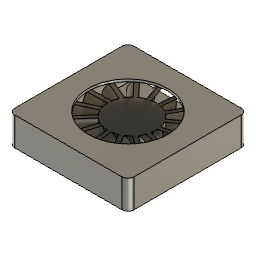
JMS583硬盘盒外壳 (Autodesk Fusion 360 archive; units mm, degrees)
design "3007涡轮风扇"
Autodesk Fusion 360 part; units mm, degrees
note: some values were not read from the file. Chosen so that the rebuilt part matches the saved one: which face or edge a step refers to; where a step ends.
box "长方体基本要素1" add length 30 width 30 height 7.2 placed x (0, 1, 0) y (-1, 0, 0) z (0, 0, 1) at (30, 0, 0) makes body 1
fillet "圆角1" radius 1.5 4 edges at (0, 0, 3.6) (30, 0, 3.6) (30, 30, 3.6) (0, 30, 3.6) on bodies 1
sketch "草图2" plane through (0, 30, 0) normal (0, 1, 0) x (-1, 0, 0)
  line L0 (-1.5, 0) -> (-1.5, 7.2)
  line L1 (-1.5, 7.2) -> (-28.5, 7.2)
  line L2 (-28.5, 7.2) -> (-28.5, 0)
  line L3 (-28.5, 0) -> (-1.5, 0)
  line L4 (-27.9, 0.6) -> (-2.1, 0.6)
  line L5 (-2.1, 0.6) -> (-2.1, 6.6)
  line L6 (-2.1, 6.6) -> (-27.9, 6.6)
  line L7 (-27.9, 6.6) -> (-27.9, 0.6)
  dimension "d10" = -0.6
extrude "拉伸1" cut sketch "草图2" against normal blind 28 contours L4 L5 L6 L7 bodies 1
sketch "草图3" plane through (0, 0, 7.2) normal (0, 0, 1) x (-1, 0, 0)
  arc A0 (-1.5, -30) -> (0, -28.5) centre (-1.5, -28.5) ccw
  line L0 (0, -28.5) -> (0, -1.5)
  arc A1 (0, -1.5) -> (-1.5, 0) centre (-1.5, -1.5) ccw
  line L1 (-1.5, 0) -> (-28.5, 0)
  arc A2 (-28.5, 0) -> (-30, -1.5) centre (-28.5, -1.5) ccw
  line L2 (-30, -1.5) -> (-30, -28.5)
  arc A3 (-30, -28.5) -> (-28.5, -30) centre (-28.5, -28.5) ccw
  line L3 (-28.5, -30) -> (-1.5, -30)
  circle A4 centre (-15, -15) radius 10
  dimension "d13" = 20
  measures "d13" diameter of A4
extrude "拉伸2" cut sketch "草图3" against normal up to surface (0.6 mm away) contours A4 bodies 1
sketch "草图4" plane through (0, 0, 0.6) normal (0, 0, 1) x (-1, 0, 0)
  line L0 (-27.9, -30) -> (-2.1, -30)
  line L1 (-2.1, -30) -> (-2.1, -2)
  line L2 (-2.1, -2) -> (-27.9, -2)
  line L3 (-27.9, -2) -> (-27.9, -30)
  circle A0 centre (-15, -15) radius 6
  dimension "d16" = 12
  measures "d16" diameter of A0
extrude "拉伸3" add sketch "草图4" along normal blind 5 separate body contours A0 makes body 2
ref_plane "工作平面1" through (15, 21, 3.0297) normal (0, 1, 0) x (1, 0, 0)
sketch "草图5" plane through (0, 21, 0) normal (0, 1, 0) x (1, 0, 0)
  line L0 (15, -7.5) -> (15, 2.5) construction
  spline S0 degree 5 poles (15, -5.6) (14.9831, -5.5891) (14.9491, -5.5667) (14.8976, -5.5318) (14.8282, -5.4822) (14.7402, -5.4155) (14.6512, -5.344) (14.5618, -5.2681) (14.473, -5.1883) (14.3862, -5.1053) (14.3029, -5.0196) (14.2243, -4.9315) (14.1513, -4.8408) (14.0838, -4.7462) (14.0213, -4.6459) (13.9629, -4.5383) (13.9079, -4.4221) (13.8562, -4.2971) (13.8086, -4.1649) (13.7665, -4.0281) (13.7316, -3.8896) (13.7053, -3.7523) (13.6885, -3.6176) (13.681, -3.4853) (13.6813, -3.3535) (13.6872, -3.2193) (13.696, -3.0801) (13.7041, -2.9338) (13.7079, -2.7799) (13.7037, -2.62) (13.6884, -2.4567) (13.6593, -2.2933) (13.6154, -2.1333) (13.557, -1.9799) (13.4868, -1.8355) (13.4089, -1.7015) (13.3279, -1.5784) (13.2483, -1.466) (13.1736, -1.3637) (13.1048, -1.2698) (13.0409, -1.1824) (12.9792, -1.0993) (12.9162, -1.0185) (12.8489, -0.9379) (12.7748, -0.8565) (12.6927, -0.7733) (12.62, -0.7051) (12.5616, -0.6529) (12.5208, -0.6177) (12.5, -0.6) knots 0 0 0 0 0 0 0.022222 0.044444 0.066667 0.088889 0.111111 0.133333 0.155556 0.177778 0.2 0.222222 0.244444 0.266667 0.288889 0.311111 0.333333 0.355556 0.377778 0.4 0.422222 0.444444 0.466667 0.488889 0.511111 0.533333 0.555556 0.577778 0.6 0.622222 0.644444 0.666667 0.688889 0.711111 0.733333 0.755556 0.777778 0.8 0.822222 0.844444 0.866667 0.888889 0.911111 0.933333 0.955556 0.977778 1 1 1 1 1 1
  spline S1 degree 3 poles (15.271, -5.1798) (15.0406, -5.0312) (14.7397, -4.7805) (14.5633, -4.5536) (14.4521, -4.4106) (14.3637, -4.2419) (14.2867, -4.0127) (14.217, -3.8056) (14.1821, -3.6167) (14.182, -3.4179) (14.1818, -3.1927) (14.2371, -2.8509) (14.1851, -2.4258) (14.1364, -2.027) (13.9458, -1.6066) (13.7657, -1.3356) (13.5507, -1.0121) (13.4347, -0.8538) (13.2399, -0.6274) (13.1243, -0.493) (12.9854, -0.3565) (12.824, -0.2192) knots 0 0 0 0 0.21724 0.21724 0.21724 0.354174 0.354174 0.354174 0.477946 0.477946 0.477946 0.618157 0.618157 0.618157 0.749718 0.749718 0.749718 0.906788 0.906788 0.906788 1 1 1 1
  spline S2 degree 5 poles (15.271, -5.1798) (15.2763, -5.1878) (15.2879, -5.2041) (15.3088, -5.229) (15.3435, -5.2633) (15.3989, -5.308) (15.4662, -5.3542) (15.5448, -5.4012) (15.6307, -5.447) (15.7206, -5.4902) (15.8127, -5.5302) (15.8872, -5.5597) (15.9435, -5.5804) (15.9811, -5.5936) (16, -5.6) knots 0 0 0 0 0 0 0.1 0.2 0.3 0.4 0.5 0.6 0.7 0.8 0.9 1 1 1 1 1 1
  line L1 (15.453, -5.3473) -> (15.6179, -5.4418)
  line L2 (16, -5.6) -> (15, -5.6)
  line L3 (12.5, -0.6) -> (13.2161, -0.6)
  point P0 (14.6, -5.3)
  point P1 (14.2, -4.9)
  point P2 (13.9, -4.4)
  point P3 (13.7, -3.7)
  point P4 (13.7, -3)
  point P5 (13.6, -2.1)
  point P6 (13.2, -1.4)
  point P7 (12.9, -1)
  point P8 (15.5354, -5.3945)
  dimension "d21" = 0.5
  constraint vertical L0
  constraint coincident L0 S0.start
  constraint midpoint P8 L1
  constraint perpendicular L0 L2
  constraint coincident S1 L3.end
  constraint horizontal L3
extrude "拉伸4" add sketch "草图5" along normal blind 5.5 separate body makes body 3
extrude "拉伸5" add 1 faces at (13.2578, 21, 1.2055) along direction (0, -1, 0) up to near side of body 2 on bodies 3 bodies 3
pattern_circular "C-阵列1" count 15 over 360 about axis through (15, 15, 0.6) along (0, 0, 1) of bodies 3 makes body 4 at (9.0269, 22.6354, 0.733) makes body 5 at (6.4377, 19.5458, 0.733) makes body 6 at (5.329, 15.6703, 0.733) makes body 7 at (3.9785, 11.9927, 1.3469) makes body 8 at (8.0308, 8.2616, 0.733) makes body 9 at (11.3741, 6.0095, 0.733) makes body 10 at (15.3443, 5.3119, 0.733) makes body 11 at (19.255, 6.2896, 0.733) makes body 12 at (22.43, 8.7733, 0.733) makes body 13 at (24.3203, 12.3337, 0.733) makes body 14 at (26.4059, 15.6501, 1.3469) makes body 15 at (23.2179, 20.1422, 0.733) makes body 16 at (20.4159, 23.0402, 0.733) makes body 17 at (16.6775, 24.5479, 0.733)
combine "合并1" operation add target body 2 tool bodies 3 4 7 10 9 8 17 15 16 14 13 12 5 11 6
sketch "草图6" plane through (0, 0, 5.6) normal (0, 0, 1) x (-1, 0, 0)
  arc A0 (-15, -21) -> (-13.5073, -20.8113) centre (-15, -15) ccw
  line L0 (-13.5073, -20.8113) -> (-11.2361, -25.9125)
  line L1 (-11.2361, -25.9125) -> (-10.3225, -25.5058)
  line L2 (-10.3225, -25.5058) -> (-12.5596, -20.4813)
  arc A1 (-12.5596, -20.4813) -> (-11.2726, -19.7018) centre (-15, -15) ccw
  line L3 (-11.2726, -19.7018) -> (-7.123, -23.4381)
  line L4 (-7.123, -23.4381) -> (-6.4538, -22.695)
  line L5 (-6.4538, -22.695) -> (-10.5411, -19.0148)
  arc A2 (-10.5411, -19.0148) -> (-9.6825, -17.7792) centre (-15, -15) ccw
  line L6 (-9.6825, -17.7792) -> (-4.3719, -19.5048)
  line L7 (-4.3719, -19.5048) -> (-4.0629, -18.5537)
  line L8 (-4.0629, -18.5537) -> (-9.2937, -16.8541)
  arc A3 (-9.2937, -16.8541) -> (-9.0118, -15.3761) centre (-15, -15) ccw
  line L9 (-9.0118, -15.3761) -> (-3.4585, -14.7924)
  line L10 (-3.4585, -14.7924) -> (-3.563, -13.7979)
  line L11 (-3.563, -13.7979) -> (-9.0329, -14.3728)
  arc A4 (-9.0329, -14.3728) -> (-9.3765, -12.908) centre (-15, -15) ccw
  line L12 (-9.3765, -12.908) -> (-4.5407, -10.116)
  line L13 (-4.5407, -10.116) -> (-5.0407, -9.25)
  line L14 (-5.0407, -9.25) -> (-9.8038, -12)
  arc A5 (-9.8038, -12) -> (-10.7136, -10.8016) centre (-15, -15) ccw
  line L15 (-10.7136, -10.8016) -> (-7.4315, -6.2841)
  line L16 (-7.4315, -6.2841) -> (-8.2405, -5.6963)
  line L17 (-8.2405, -5.6963) -> (-11.4733, -10.1459)
  arc A6 (-11.4733, -10.1459) -> (-12.7918, -9.4211) centre (-15, -15) ccw
  line L18 (-12.7918, -9.4211) -> (-11.6309, -3.9592)
  line L19 (-11.6309, -3.9592) -> (-12.609, -3.7513)
  line L20 (-12.609, -3.7513) -> (-13.7525, -9.1311)
  arc A7 (-13.7525, -9.1311) -> (-15.2519, -9.0053) centre (-15, -15) ccw
  line L21 (-15.2519, -9.0053) -> (-16.4128, -3.5434)
  line L22 (-16.4128, -3.5434) -> (-17.391, -3.7513)
  line L23 (-17.391, -3.7513) -> (-16.2475, -9.1311)
  arc A8 (-16.2475, -9.1311) -> (-17.6684, -9.626) centre (-15, -15) ccw
  line L24 (-17.6684, -9.626) -> (-20.9505, -5.1085)
  line L25 (-20.9505, -5.1085) -> (-21.7595, -5.6963)
  line L26 (-21.7595, -5.6963) -> (-18.5267, -10.1459)
  arc A9 (-18.5267, -10.1459) -> (-19.6235, -11.1759) centre (-15, -15) ccw
  line L27 (-19.6235, -11.1759) -> (-24.4593, -8.384)
  line L28 (-24.4593, -8.384) -> (-24.9593, -9.25)
  line L29 (-24.9593, -9.25) -> (-20.1962, -12)
  arc A10 (-20.1962, -12) -> (-20.7791, -13.3871) centre (-15, -15) ccw
  line L30 (-20.7791, -13.3871) -> (-26.3325, -12.8034)
  line L31 (-26.3325, -12.8034) -> (-26.437, -13.7979)
  line L32 (-26.437, -13.7979) -> (-20.9671, -14.3728)
  arc A11 (-20.9671, -14.3728) -> (-20.9355, -15.8771) centre (-15, -15) ccw
  line L33 (-20.9355, -15.8771) -> (-26.2462, -17.6026)
  line L34 (-26.2462, -17.6026) -> (-25.9372, -18.5537)
  line L35 (-25.9372, -18.5537) -> (-20.7063, -16.8541)
  arc A12 (-20.7063, -16.8541) -> (-20.0656, -18.2155) centre (-15, -15) ccw
  line L36 (-20.0656, -18.2155) -> (-24.2153, -21.9519)
  line L37 (-24.2153, -21.9519) -> (-23.5462, -22.695)
  line L38 (-23.5462, -22.695) -> (-19.4589, -19.0148)
  arc A13 (-19.4589, -19.0148) -> (-18.3198, -19.9979) centre (-15, -15) ccw
  line L39 (-18.3198, -19.9979) -> (-20.591, -25.099)
  line L40 (-20.591, -25.099) -> (-19.6775, -25.5058)
  line L41 (-19.6775, -25.5058) -> (-17.4404, -20.4813)
  arc A14 (-17.4404, -20.4813) -> (-16, -20.9161) centre (-15, -15) ccw
  line L42 (-16, -20.9161) -> (-16, -26.5)
  line L43 (-16, -26.5) -> (-15, -26.5)
  line L44 (-15, -26.5) -> (-15, -21)
  circle A15 centre (-15, -15) radius 11
  circle A16 centre (-15, -15) radius 9
  line L45 (0, 0) -> (-30, 0)
  line L46 (-30, 0) -> (-30, -30)
  line L47 (-30, -30) -> (0, -30)
  line L48 (0, -30) -> (0, 0)
  line L49 (0, 0) -> (-30, -30) construction
  line L50 (-30, 0) -> (0, -30) construction
  point P0 (-15, -15)
  dimension "d28" = 22
  dimension "d29" = 18
  constraint concentric A0 A15
  constraint concentric A0 A16
  constraint horizontal L45
  constraint perpendicular L45 L46
  constraint parallel L45 L47
  constraint parallel L46 L48
  constraint coincident L49 P0
  constraint coincident L50 P0
  constraint coincident L45.start L48.end
  constraint coincident P0 A0.centre
  measures "d28" diameter of A15
  measures "d29" diameter of A16
extrude "拉伸6" cut sketch "草图6" against normal up to surface (5 mm away) contours L42 L43 L44 A15 | L0 L1 L2 A15 | L39 L40 L41 A15 | L3 L4 L5 A15 | L36 L37 L38 A15 | L6 L7 L8 A15 | L33 L34 L35 A15 | L9 L10 L11 A15 | L30 L31 L32 A15 | L12 L13 L14 A15 | L27 L28 L29 A15 | L15 L16 L17 A15 | L24 L25 L26 A15 | L18 L19 L20 A15 | L21 L22 L23 A15 | L45 L46 L47 L48 bodies 2
copy_body "实体->零部件1" bodies 1 removing the originals makes body 18 in component "涡轮风扇外壳"
copy_body "实体->零部件2" bodies 2 removing the originals makes body 19 in component "扇叶"
component "扇叶" placed x (1, 0, 0) y (0, 1, 0) z (0, 0, 1) at (0, 1, 0)
component "涡轮风扇外壳" placed x (1, 0, 0) y (0, 1, 0) z (0, 0, 1) at (0, 0, 0)
named bodies: "涡轮风扇外壳", "扇叶"
